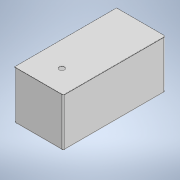
# Autodesk Inventor part: oil_water_separator
Saved by Autodesk Inventor 2020 (Build 240168000, 168)
## iProperties
Created: 2022-08-31
Part Number: oil_water_separator
Material: Generic
Document SubType Name: Modeling
Designer: Intuito_PC
Density: 1 g/cm^3
Appearance: Default
Author: Intuito_PC
Autodesk Inventor part; units mm, degrees
ref_plane "YZ Plane" through (0, 0, 0) normal (1, 0, 0) x (0, 1, 0)
ref_plane "XZ Plane" through (0, 0, 0) normal (0, 1, 0) x (-1, 0, 0)
ref_plane "XY Plane" through (0, 0, 0) normal (0, 0, 1) x (1, 0, 0)
sketch "Sketch1" plane through (0, 0, 0) normal (0, 0, 1) x (1, 0, 0)
  line L0 (0, 0) -> (-110, 0)
  line L1 (-110, 0) -> (-110, 110)
  line L2 (-110, 110) -> (0, 110)
  line L3 (0, 110) -> (0, 0)
  dimension "d0" = 110
  dimension "d1" = 110
  constraints: 8 end point, 2 parallel, 1 horizontal, 1 perpendicular
  measures "d0" distance of L1.end L2.end
  measures "d1" distance of L0.end L1.end
extrude "Extrusion1" add sketch "Sketch1" along normal blind 230
fillet "Fillet2" radius 3.175 8 edges at (-110, 55, 230) (0, 55, 230) (-55, 0, 230) (-110, 0, 115) (0, 0, 115) (0, 55, 0) (-55, 0, 0) (-110, 55, 0)
shell "Shell1" thickness 0.5 removed faces 1 at (-36.6667, 110, 77.725)
sketch "Sketch2" plane through (-106.825, 110, 0) normal (0, 1, 0) x (1, 0, 0)
  line L0 (-2.54, -230.635) -> (107.9059, -230.635)
  line L1 (107.9059, -230.635) -> (107.9059, -0.635)
  line L2 (107.9059, -0.635) -> (-2.54, -0.635)
  line L3 (-2.54, -0.635) -> (-2.54, -230.635)
  point P0 (106.825, 0)
  point P1 (0, -229.5)
  point P2 (103.65, -3.175)
  dimension "d11" = 230
  constraints: 8 end point, 2 parallel, 1 perpendicular
  measures "d11" distance of L2.end L0.start
extrude "Extrusion2" add sketch "Sketch2" along normal blind 0.5
fillet "Fillet4" radius 3.175 2 edges at (1.0809, 110.25, 230.635) (1.0809, 110.25, 0.635)
sketch "Sketch3" plane through (-106.825, 110.5, 0) normal (0, 1, 0) x (1, 0, 0)
  point P0 (106.825, 0)
  point P1 (53.8726, -180.2016)
hole "Hole1" at (-52.9524, 110.5, 180.2016) direction (0, -1, 0) diameter 12 depth 10 tip angle 118
sketch "Sketch4" plane through (-106.825, 0, 3.175) normal (0, -1, 0) x (1, 0, 0)
  point P0 (106.825, -3.175)
  point P1 (53.016, 39.15)
hole "Hole2" at (-53.809, 0, 42.325) direction (0, 1, 0) diameter 18 depth 10 tip angle 118
sketch "Sketch5" plane through (-106.825, 0, 3.175) normal (0, -1, 0) x (1, 0, 0)
  circle A0 centre (53.016, 39.15) radius 9 projected
  circle A1 centre (53.016, 39.15) radius 10
  point P0 (106.825, -3.175)
  dimension "d27" = 20
  constraints: 1 centre point, 1 coincident
  measures "d27" diameter of A1
extrude "Extrusion3" add sketch "Sketch5" along normal blind 40 contours A0 | A1
sketch "Sketch6" plane through (-53.809, -40, 42.325) normal (0, -1, 0) x (1, 0, 0)
  point P0 (53.809, -42.325)
  point P1 (0.11, 0.0758)
hole "Hole3" at (-53.6991, -40, 42.4008) direction (0, 1, 0) diameter 18 depth 10 tip angle 118
body "Solid1"
